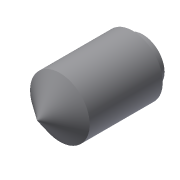
# Autodesk Inventor part: 00_Olympus_40_1.3oil
Saved by Autodesk Inventor 2019.4 (Build 234330000, 330)
## iProperties
Created: 2021-01-12
Part Number: 00_Olympus_40_1.3oil
Material: Generic
Document SubType Name: Modeling
Designer: diederichbenedict
Density: 1 g/cm^3
Appearance: Default
Author: diederichbenedict
Autodesk Inventor part; units mm, degrees
ref_plane "YZ Plane" through (0, 0, 0) normal (1, 0, 0) x (0, 1, 0)
ref_plane "XZ Plane" through (0, 0, 0) normal (0, 1, 0) x (-1, 0, 0)
ref_plane "XY Plane" through (0, 0, 0) normal (0, 0, 1) x (1, 0, 0)
sketch "Sketch1" plane through (0, 0, 0) normal (1, 0, 0) x (0, 1, 0)
  line L0 (0, 0) -> (0, 49.7)
  line L1 (0, 0) -> (49.7, 0) construction
  line L2 (0, 49.7) -> (14, 39)
  line L3 (14, 39) -> (14, 4.7)
  line L4 (14, 4.7) -> (10.16, 4.7)
  line L5 (10.16, 4.7) -> (10.16, 0)
  line L6 (10.16, 0) -> (0, 0)
  dimension "d0" = 49.7
  dimension "d1" = 90
  dimension "d2" = 10.16
  dimension "d3" = 14
  dimension "d4" = 39
  dimension "d5" = 4.7
  constraints: 14 end point, 4 perpendicular, 1 horizontal, 1 parallel, 1 vertical
  measures "d0" distance of L0.start L0.end
  measures "d1" angle of L1 L0
  measures "d2" distance between parallel lines of L0 L5
  measures "d3" distance between parallel lines of L0 L3
  measures "d4" distance from line of L1 L2.end
  measures "d5" distance between parallel lines of L1 L4
revolve "Revolution1" add sketch "Sketch1" angle 360 about axis through (0, 0, 0) along (0, 0, 1)
body "Solid1"
